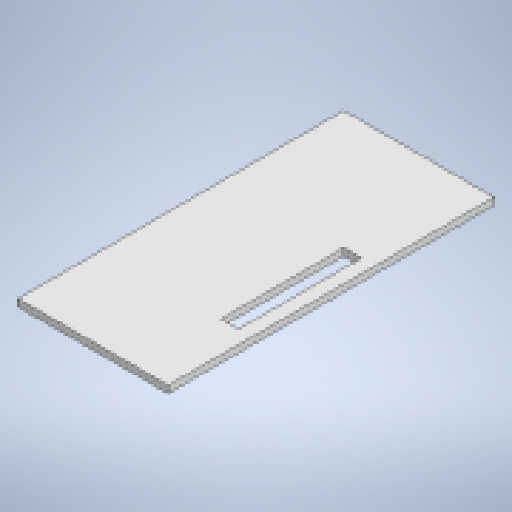
# Autodesk Inventor part: Arduino Lid
Saved by Autodesk Inventor 2024 (Build 280153000, 153)
## iProperties
Created: 2023-11-29
Part Number: Arduino Lid
Material: Generic
Document SubType Name: Modeling
Designer: close
Density: 1 g/cm^3
Appearance: Default
Author: close
Autodesk Inventor part; units mm, degrees
ref_plane "YZ Plane" through (0, 0, 0) normal (1, 0, 0) x (0, 1, 0)
ref_plane "XZ Plane" through (0, 0, 0) normal (0, 1, 0) x (-1, 0, 0)
ref_plane "XY Plane" through (0, 0, 0) normal (0, 0, 1) x (1, 0, 0)
sketch "Sketch1" plane through (0, 0, 0) normal (0, 1, 0) x (-1, 0, 0)
  line L0 (20.49, -1.25) -> (1.25, -1.25)
  line L1 (1.25, -1.25) -> (1.25, -45.89)
  line L2 (1.25, -45.89) -> (20.49, -45.89)
  line L3 (20.49, -45.89) -> (20.49, -1.25)
  line L4 (18.49, -3.25) -> (3.25, -3.25) construction
  line L5 (3.25, -3.25) -> (3.25, -43.89) construction
  line L6 (3.25, -43.89) -> (18.49, -43.89) construction
  line L7 (18.49, -43.89) -> (18.49, -3.25) construction
  circle A0 centre (18.49, -3.25) radius 2 construction
  circle A1 centre (18.49, -3.25) radius 0.75 construction
  circle A2 centre (18.49, -43.89) radius 2 construction
  circle A3 centre (18.49, -43.89) radius 0.75 construction
  circle A4 centre (3.25, -43.89) radius 2 construction
  circle A5 centre (3.25, -43.89) radius 0.75 construction
  circle A6 centre (3.25, -3.25) radius 2 construction
  circle A7 centre (3.25, -3.25) radius 0.75 construction
  line L8 (0, -47.14) -> (21.74, -47.14)
  line L9 (21.74, -47.14) -> (21.74, 0)
  line L10 (21.74, 0) -> (0, 0)
  line L11 (0, 0) -> (0, -47.14)
  line L12 (19.49, -2.25) -> (2.25, -2.25)
  line L13 (2.25, -2.25) -> (2.25, -44.89)
  line L14 (2.25, -44.89) -> (19.49, -44.89)
  line L15 (19.49, -44.89) -> (19.49, -2.25)
  dimension "d2" = 40.64
  dimension "d3" = 15.24
  dimension "d4" = 1.5
  dimension "d5" = 4
  dimension "d6" = 1.25
  dimension "d7" = 1.25
  dimension "d8" = 1.25
  dimension "d9" = 1.25
  dimension "d12" = 1
  dimension "d13" = 1
  dimension "d14" = 1
  dimension "d15" = 1
  constraints: 32 end point, 9 coincident, 8 centre point, 8 parallel, 6 equal radius, 4 horizontal, 4 perpendicular, 4 tangent
  measures "d2" distance of L7.start L7.end
  measures "d3" distance of L7.end L5.start
  measures "d4" diameter of A1
  measures "d5" diameter of A0
  measures "d6" distance between parallel lines of L3 L9
  measures "d7" distance between parallel lines of L10 L0
  measures "d8" distance between parallel lines of L8 L2
  measures "d9" distance between parallel lines of L1 L11
  measures "d12" distance between parallel lines of L15 L3
  measures "d13" distance between parallel lines of L0 L12
  measures "d14" distance between parallel lines of L1 L13
  measures "d15" distance between parallel lines of L2 L14
extrude "Extrusion1" add sketch "Sketch1" against normal blind 1 contours L3 L2 L1 L0
extrude "Extrusion2" add sketch "Sketch1" along normal blind 1 contours L3 L2 L1 L0 | L11 L10 L9 L8 | L15 L14 L13 L12
sketch "Sketch2" plane through (0, -1, 0) normal (0, -1, 0) x (1, 0, 0)
  line L0 (-4.52, -29.92) -> (-1.98, -29.92)
  line L1 (-1.98, -29.92) -> (-1.98, -12.14)
  line L2 (-1.98, -12.14) -> (-4.52, -12.14)
  line L3 (-4.52, -12.14) -> (-4.52, -29.92)
  circle A0 centre (-3.25, -28.65) radius 0.508 construction
  circle A1 centre (-3.25, -13.41) radius 0.508 construction
  point P0 (0, 0)
  point P1 (-3.25, -29.92)
  dimension "d20" = 2.54
  dimension "d21" = 17.78
  dimension "d22" = 15.24
  dimension "d23" = 1.27
  dimension "d24" = 1.27
  constraints: 8 end point, 2 parallel, 1 horizontal, 1 midpoint, 1 perpendicular
  measures "d20" distance between parallel lines of L1 L3
  measures "d21" distance between parallel lines of L2 L0
  measures "d22" distance of A1.centre A0.centre
  measures "d23" distance of point (-3.25, -29.92) A0.centre
  measures "d24" distance from line of L3 A1.centre
extrude "Extrusion3" cut sketch "Sketch2" against normal through all
equation "\"d7\" = d6"
equation "\"d8\" = d7"
equation "\"d9\" = d7"
equation "\"d21\" = 7 * d20"
equation "\"d23\" = -0.5 * d22 + 0.5 * d21"
equation "\"d24\" = 0.5 * d20"
body "Solid1"
